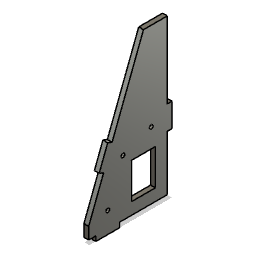
monitor_stand_plate (Autodesk Fusion 360 design; units mm, degrees)
Autodesk Fusion 360 part; units mm, degrees
note: some values were not read from the file. Set by a fixed rule: the direction of a hole.
sketch "スケッチ1" plane through (0, 0, 0) normal (1, 0, 0) x (0, 0, -1)
  line L0 (0, 0) -> (-66, 0)
  line L1 (-66, 0) -> (-66, 10)
  line L2 (-66, 10) -> (-20, 130)
  line L3 (-20, 130) -> (0, 130)
  line L4 (0, 130) -> (0, 0)
  line L5 (-40, 0) -> (-60, 0)
  line L6 (-60, 0) -> (-60, -4)
  line L7 (-60, -4) -> (-40, -4)
  line L8 (-40, -4) -> (-40, 0)
  line L9 (0, 46) -> (4, 46)
  line L10 (4, 46) -> (4, 66)
  line L11 (4, 66) -> (0, 66)
  line L12 (0, 66) -> (0, 46)
  line L13 (-50, 0) -> (-50, 13.5)
  line L14 (0, 56) -> (-13.5, 56)
  line L15 (-53.4722, 42.6811) -> (-46.3135, 61.356)
  line L16 (-46.3135, 61.356) -> (-50.0485, 62.7878)
  line L17 (-50.0485, 62.7878) -> (-57.2072, 44.1129)
  line L18 (-57.2072, 44.1129) -> (-53.4722, 42.6811)
  line L19 (-49.8929, 52.0186) -> (-37.2873, 47.1864)
  line L20 (-10, 10) -> (-30, 10)
  line L21 (-30, 10) -> (-30, 40)
  line L22 (-30, 40) -> (-10, 40)
  line L23 (-10, 40) -> (-10, 10)
  dimension "d1" = 66
  dimension "d2" = 10
  dimension "d5" = 130
  dimension "d6" = 20
  dimension "d7" = 4
  dimension "d8" = 20
  dimension "d9" = 46
  dimension "d10" = 20
  dimension "d11" = 4
  dimension "d12" = 40
  dimension "d13" = 20
  dimension "d14" = 4
  dimension "d15" = 35
  dimension "d16" = 13.5
  dimension "d22" = 10
  dimension "d23" = 20
  dimension "d24" = 10
  dimension "d25" = 30
  constraint coincident L0.start L4.end
  constraint horizontal L0
  constraint perpendicular L0 L1
  constraint parallel L0 L3
  constraint perpendicular L0 L4
  constraint horizontal L5
  constraint vertical L6
  constraint horizontal L7
  constraint vertical L8
  constraint coincident L0 L5.start
  constraint horizontal L9
  constraint vertical L10
  constraint horizontal L11
  constraint vertical L12
  constraint coincident L4 L9.start
  constraint midpoint L5 L13.start
  constraint perpendicular L0 L13
  constraint midpoint L12 L14.start
  constraint perpendicular L4 L14
  constraint perpendicular L15 L16
  constraint parallel L15 L17
  constraint parallel L16 L18
  constraint coincident L2 L15.end
  constraint parallel L2 L15
  constraint midpoint L15 L19.start
  constraint perpendicular L2 L19
  constraint equal L14 L19
  constraint equal L13 L19
  constraint horizontal L20
  constraint vertical L21
  constraint horizontal L22
  constraint vertical L23
  measures "d1" distance of L0.start L0.end
  measures "d2" distance of L0.end L1.end
  measures "d5" distance of L3.end L0.start
  measures "d6" distance of L2.end L3.end
  measures "d7" distance of L10.end L11.end
  measures "d8" distance of L9.end L10.end
  measures "d9" distance of L0.start L9
  measures "d10" distance of L6.end L7.end
  measures "d11" distance of L5.end L6.end
  measures "d12" distance of L0.start L8
  measures "d13" distance of L16.end L17.end
  measures "d14" distance of L15.end L16.end
  measures "d15" distance of L1.end L15.start
  measures "d16" distance of L19.start L19.end
  measures "d22" distance of L0.start L23
  measures "d23" distance of L21.end L22.end
  measures "d24" distance of L0 L20
  measures "d25" distance of L20.end L21.end
extrude "押し出し1" add sketch "スケッチ1" along normal blind 4
hole "穴1" at (0, 56, 13.5) at (0, 47.1864, 37.2873) at (0, 13.5, 50) direction (1, 0, 0) diameter 3.2 end through all
